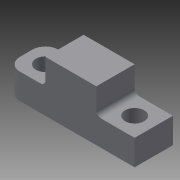
# Autodesk Inventor part: Mirror
Saved by Autodesk Inventor 2015 (Build 190159000, 159)
## iProperties
Created: 2015-02-24
Part Number: Mirror
Material: Generic
Document SubType Name: Modeling
Designer: PLTW-Stu-02
Density: 1 g/cm^3
Appearance: Default
Author: PLTW-Stu-02
Autodesk Inventor part; units mm, degrees
ref_plane "YZ Plane" through (0, 0, 0) normal (1, 0, 0) x (0, 1, 0)
ref_plane "XZ Plane" through (0, 0, 0) normal (0, 1, 0) x (-1, 0, 0)
ref_plane "XY Plane" through (0, 0, 0) normal (0, 0, 1) x (1, 0, 0)
sketch "Sketch1" plane through (0, 0, 0) normal (0, 0, 1) x (1, 0, 0)
  line L0 (43.4638, 27.4592) -> (30.7638, 27.4592)
  line L1 (30.7638, 27.4592) -> (30.7638, 14.7592)
  line L2 (43.4638, 14.7592) -> (43.4638, 27.4592)
  line L3 (30.7638, 14.7592) -> (11.7138, 14.7592)
  line L4 (11.7138, 14.7592) -> (11.7138, 2.0592)
  line L5 (11.7138, 2.0592) -> (43.4638, 2.0592)
  line L6 (43.4638, 2.0592) -> (43.4638, 14.7592)
  point P0 (0, 0)
  dimension "d1" = 12.7
  dimension "d2" = 31.75
  dimension "d3" = 12.7
  constraints: 14 end point, 3 parallel, 2 horizontal, 2 perpendicular
  measures "d1" distance of L1.end L0.end
  measures "d2" distance of L5.end L4.end
  measures "d3" distance of L4.end L3.end
extrude "Extrusion1" add sketch "Sketch1" along normal blind 19.05
fillet "Fillet1" radius 6.35 2 edges at (11.7138, 8.4092, 19.05) (11.7138, 8.4092, 0)
sketch "Sketch2" plane through (30.7638, 14.7592, 19.05) normal (0, 1, 0) x (1, 0, 0)
  circle A0 centre (-9.525, 9.525) radius 4.7625
  point P0 (-30.7638, 19.05)
  point P1 (-31.0867, 15.9672)
  dimension "d8" = 9.525
  constraints: 1 centre point, 1 coincident
  measures "d8" diameter of A0
hole "Hole1" at (21.2388, 14.7592, 9.525) at (-0.3229, 14.7592, 3.0828) at (21.2388, 14.7592, 9.525) direction (0, -1, 0) diameter 9.525 depth 25.4 tip angle 118
sketch "Sketch4" plane through (0, 0, 19.05) normal (0, 0, 1) x (1, 0, 0)
  line L0 (75.2138, 14.7592) -> (75.2138, 2.0592)
  line L1 (75.2138, 2.0592) -> (43.4638, 2.0592)
  line L2 (43.4638, 2.0592) -> (43.4638, 27.4592)
  line L3 (43.4638, 27.4592) -> (56.1638, 27.4592)
  line L4 (56.1638, 27.4592) -> (56.1638, 14.7592)
  line L5 (56.1638, 14.7592) -> (75.2138, 14.7592)
  point P0 (0, 0)
  dimension "d16" = 31.75
  dimension "d17" = 12.7
  constraints: 12 end point, 1 parallel, 1 vertical
  measures "d16" distance of L0.end L1.end
  measures "d17" distance of L2.end L3.end
extrude "Extrusion3" add sketch "Sketch4" against normal blind 19.05
sketch "Sketch6" plane through (56.1638, 14.7592, 19.05) normal (0, 1, 0) x (1, 0, 0)
  line L0 (-38.1, 19.05) -> (19.05, 19.05) projected
  point P0 (-56.1638, 19.05)
  point P1 (9.525, 9.525)
hole "Hole2" at (65.6888, 14.7592, 9.525) direction (0, -1, 0) diameter 9.525 end through all
fillet "Fillet4" radius 2.54 1 edges at (30.7638, 14.7592, 9.525)
fillet "Fillet5" radius 2.54 1 edges at (56.1638, 14.7592, 9.525)
body "Solid1"
